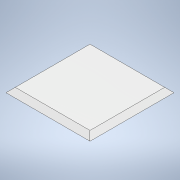
# Autodesk Inventor part: Base Plate
Saved by Autodesk Inventor 2021.1 (Build 251245010, 245A)
## iProperties
Created: 2020-11-23
Part Number: Base Plate
Material: PC/ABS Plastic
Document SubType Name: Modeling
Designer: elizh
Density: 0.357273 g/cm^3
Appearance: Smooth - White
Author: elizh
Autodesk Inventor part; units mm, degrees
ref_plane "YZ Plane" through (0, 0, 0) normal (1, 0, 0) x (0, 1, 0)
ref_plane "XZ Plane" through (0, 0, 0) normal (0, 1, 0) x (-1, 0, 0)
ref_plane "XY Plane" through (0, 0, 0) normal (0, 0, 1) x (1, 0, 0)
sketch "Sketch1" plane through (0, 0, 0) normal (0, 1, 0) x (-1, 0, 0)
  line L0 (45, 45) -> (-45, 45)
  line L1 (-45, 45) -> (-45, -45)
  line L2 (-45, -45) -> (45, -45)
  line L3 (45, -45) -> (45, 45)
  line L4 (0, 0) -> (55.2623, 0) construction
  line L5 (0, 0) -> (0, -72.148) construction
  dimension "d0" = 90
  constraints: 12 end point, 2 horizontal, 2 parallel, 2 perpendicular, 1 vertical, 2 other
  measures "d0" distance of L2.end L0.start
extrude "Extrusion1" add sketch "Sketch1" along normal blind 5
chamfer "Chamfer2" distance 5 angle 45 4 edges at (-45, 5, 0) (0, 5, -45) (45, 5, 0) (0, 5, 45)
body "Solid1"
